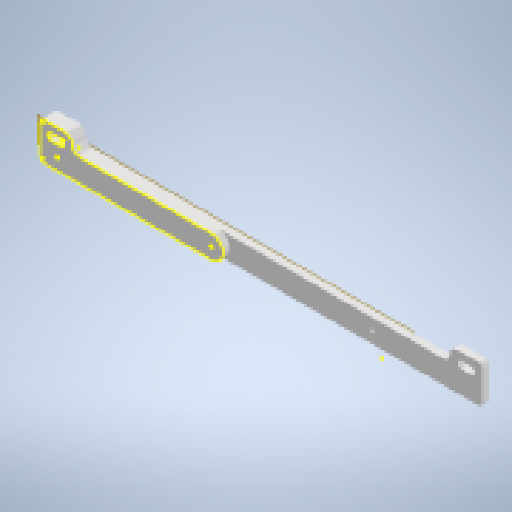
# Autodesk Inventor part: divider
Saved by Autodesk Inventor 2023 (Build 270158000, 158)
## iProperties
Created: 2022-09-07
Part Number: divider
Material: Generic
Document SubType Name: Modeling
Designer: grant
Density: 1 g/cm^3
Appearance: Default
Author: grant
Autodesk Inventor part; units mm, degrees
ref_plane "YZ Plane" through (0, 0, 0) normal (1, 0, 0) x (0, 1, 0)
ref_plane "XZ Plane" through (0, 0, 0) normal (0, 1, 0) x (-1, 0, 0)
ref_plane "XY Plane" through (0, 0, 0) normal (0, 0, 1) x (1, 0, 0)
ref_plane "Work Plane1" through (0, 0, 0) normal (0, 0, 1) x (1, 0, 0)
sketch "Sketch1" plane through (0, 0, 0) normal (0, 0, 1) x (1, 0, 0)
  circle A0 centre (-15, 10) radius 1.6 projected
  circle A1 centre (-285, 10) radius 1.6 projected
  circle A2 centre (-285, 10) radius 1.6 projected
  circle A3 centre (-150, 10) radius 1.6 projected
  circle A4 centre (-15, 10) radius 1.6 projected
  line L0 (0, 0) -> (0, 20) projected
  line L1 (0, 20) -> (-300, 20) projected
  line L2 (-300, 0) -> (-300, 20) projected
  line L3 (0, 0) -> (-300, 0) projected
  line L4 (-300, 20) -> (81, 20)
  line L5 (81, 20) -> (81, 0)
  line L6 (81, 0) -> (-300, 0)
  line L7 (-300, 0) -> (-300, 20)
  point P0 (81, 10)
  point P1 (-300, 10)
  dimension "d0" = 381
  constraints: 8 end point, 2 midpoint, 2 parallel, 1 horizontal, 1 perpendicular
  measures "d0" distance of point (81, 10) point (-300, 10)
extrude "Extrusion1" add sketch "Sketch1" along normal blind 6.35
sketch "Sketch2" plane through (0, 0, 6.35) normal (0, 0, 1) x (1, 0, 0)
  line L0 (81, 20) -> (-300, 20) projected
  line L1 (-300, 20) -> (-300, 0) projected
  line L2 (-300, 0) -> (81, 0) projected
  line L3 (81, 0) -> (81, 20) projected
  circle A0 centre (-150, 10) radius 1.6 projected
  circle A1 centre (-285, 10) radius 1.6 projected
  circle A2 centre (-15, 10) radius 1.6 projected
  line L4 (81, 20) -> (53.06, 20)
  line L5 (53.06, 20) -> (53.06, 32.7)
  line L6 (53.06, 32.7) -> (81, 32.7)
  line L7 (81, 32.7) -> (81, 20)
  line L8 (74.65, 20) -> (59.41, 20)
  line L9 (59.41, 20) -> (59.41, 26.35)
  line L10 (59.41, 26.35) -> (74.65, 26.35)
  line L11 (74.65, 26.35) -> (74.65, 20)
  line L12 (-278.41, 20) -> (-293.65, 20)
  line L13 (-272.06, 20) -> (-300, 20)
  line L14 (-278.41, 26.35) -> (-278.41, 20)
  line L15 (-293.65, 20) -> (-293.65, 26.35)
  line L16 (-293.65, 26.35) -> (-278.41, 26.35)
  line L17 (-300, 20) -> (-300, 32.7)
  line L18 (-300, 32.7) -> (-272.06, 32.7)
  line L19 (-272.06, 32.7) -> (-272.06, 20)
  point P0 (0, 0)
  point P1 (74.65, 23.175)
  point P2 (67.03, 32.7)
  point P3 (-278.41, 23.175)
  point P4 (-286.03, 32.7)
  dimension "d3" = 6.35
  dimension "d4" = 6.35
  dimension "d5" = 6.35
  dimension "d6" = 15.24
  dimension "d7" = 6.35
  dimension "d10" = 353.06
  constraints: 32 end point, 4 parallel, 3 horizontal, 2 midpoint, 2 perpendicular, 2 point on line, 18 other
  measures "d3" distance from line of point (74.65, 23.175) L7
  measures "d4" distance between parallel lines of L5 L9
  measures "d5" distance from line of point (67.03, 32.7) L10
  measures "d6" distance between parallel lines of L9 L11
  measures "d7" distance between parallel lines of L10 L0
  measures "d10" distance of L8.end L12.end
extrude "Extrusion2" add sketch "Sketch2" against normal blind 6.35 contours L0 L11 L10 L9 L5 L6 L7 | L17 L18 L19 L0 L14 L16 L15
fillet "Fillet1" radius 6.35 4 edges at (53.06, 20, 3.175) (-272.06, 20, 3.175) (-272.06, 32.7, 3.175) (53.06, 32.7, 3.175)
fillet "Fillet2" radius 3.175 12 edges at (-278.41, 20, 3.175) (-278.41, 26.35, 3.175) (-293.65, 20, 3.175) (-293.65, 26.35, 3.175) (-300, 32.7, 3.175) (-300, 0, 3.175) (81, 0, 3.175) (81, 32.7, 3.175) (59.41, 26.35, 3.175) (59.41, 20, 3.175) (74.65, 20, 3.175) (74.65, 26.35, 3.175)
sketch "Sketch3" plane through (0, 0, 6.35) normal (0, 0, 1) x (1, 0, 0)
  arc A0 (81, 29.525) -> (77.825, 32.7) centre (77.825, 29.525) ccw projected
  line L0 (77.825, 32.7) -> (59.41, 32.7) projected
  arc A1 (59.41, 32.7) -> (53.06, 26.35) centre (59.41, 26.35) ccw projected
  arc A2 (46.71, 20) -> (53.06, 26.35) centre (46.71, 26.35) ccw projected
  line L1 (46.71, 20) -> (-265.71, 20) projected
  arc A3 (-272.06, 26.35) -> (-265.71, 20) centre (-265.71, 26.35) ccw projected
  arc A4 (-272.06, 26.35) -> (-278.41, 32.7) centre (-278.41, 26.35) ccw projected
  line L2 (-278.41, 32.7) -> (-296.825, 32.7) projected
  arc A5 (-296.825, 32.7) -> (-300, 29.525) centre (-296.825, 29.525) ccw projected
  line L3 (-300, 29.525) -> (-300, 3.175) projected
  arc A6 (-300, 3.175) -> (-296.825, 0) centre (-296.825, 3.175) ccw projected
  line L4 (-296.825, 0) -> (77.825, 0) projected
  arc A7 (77.825, 0) -> (81, 3.175) centre (77.825, 3.175) ccw projected
  line L5 (81, 3.175) -> (81, 29.525) projected
  arc A8 (62.585, 26.35) -> (62.585, 20) centre (62.585, 23.175) ccw projected
  line L6 (62.585, 26.35) -> (71.475, 26.35) projected
  arc A9 (71.475, 20) -> (71.475, 26.35) centre (71.475, 23.175) ccw projected
  line L7 (71.475, 20) -> (62.585, 20) projected
  line L8 (-290.475, 26.35) -> (-281.585, 26.35) projected
  arc A10 (-281.585, 20) -> (-281.585, 26.35) centre (-281.585, 23.175) ccw projected
  line L9 (-281.585, 20) -> (-290.475, 20) projected
  arc A11 (-290.475, 26.35) -> (-290.475, 20) centre (-290.475, 23.175) ccw projected
  circle A12 centre (-150, 10) radius 1.6 projected
  circle A13 centre (-285, 10) radius 1.6 projected
  circle A14 centre (-15, 10) radius 1.6 projected
  circle A15 centre (-150, 10) radius 10
  point P0 (0, 0)
  point P1 (-150, 0)
  point P2 (-150, 20)
  constraints: 1 centre point, 1 coincident, 1 tangent
extrude "Extrusion3" add sketch "Sketch3" along normal blind 6.35 contours L4 A6 L3 A5 L2 A4 A3 L1 A15 | A15
sketch "Sketch4" plane through (0, 0, 12.7) normal (0, 0, 1) x (1, 0, 0)
  line L0 (-150, 20) -> (-265.71, 20) projected
  arc A0 (-272.06, 26.35) -> (-265.71, 20) centre (-265.71, 26.35) ccw projected
  arc A1 (-272.06, 26.35) -> (-278.41, 32.7) centre (-278.41, 26.35) ccw projected
  line L1 (-278.41, 32.7) -> (-296.825, 32.7) projected
  arc A2 (-296.825, 32.7) -> (-300, 29.525) centre (-296.825, 29.525) ccw projected
  line L2 (-300, 29.525) -> (-300, 3.175) projected
  arc A3 (-300, 3.175) -> (-296.825, 0) centre (-296.825, 3.175) ccw projected
  line L3 (-296.825, 0) -> (-150, 0) projected
  arc A4 (-150, 0) -> (-150, 20) centre (-150, 10) ccw projected
  line L4 (-281.585, 20) -> (-290.475, 20) projected
  arc A5 (-290.475, 26.35) -> (-290.475, 20) centre (-290.475, 23.175) ccw projected
  line L5 (-290.475, 26.35) -> (-281.585, 26.35) projected
  arc A6 (-281.585, 20) -> (-281.585, 26.35) centre (-281.585, 23.175) ccw projected
  circle A7 centre (-285, 10) radius 1.6 projected
  circle A8 centre (-150, 10) radius 1.6 projected
  point P0 (0, 0)
body "Solid1"
